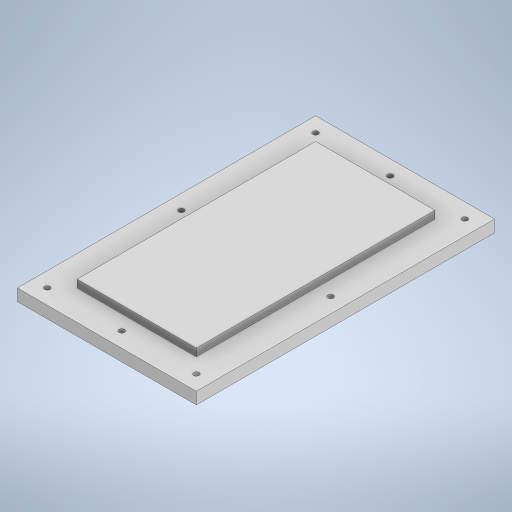
# Autodesk Inventor part: Faceplate
Saved by Autodesk Inventor 2024 (Build 280153020, 153B)
## iProperties
Created: 2023-07-16
Part Number: Faceplate
Material: Generic
Document SubType Name: Modeling
Designer: torban
Density: 1 g/cm^3
Appearance: Default
Author: torban
Autodesk Inventor part; units mm, degrees
ref_plane "YZ Plane" through (0, 0, 0) normal (1, 0, 0) x (0, 1, 0)
ref_plane "XZ Plane" through (0, 0, 0) normal (0, 1, 0) x (-1, 0, 0)
ref_plane "XY Plane" through (0, 0, 0) normal (0, 0, 1) x (1, 0, 0)
sketch "Sketch1" plane through (0, 0, 0) normal (0, 1, 0) x (-1, 0, 0)
  line L0 (0, 0) -> (100, 0)
  line L1 (100, 0) -> (100, -200)
  line L2 (100, -200) -> (0, -200)
  line L3 (0, -200) -> (0, 0)
  dimension "d0" = 200
  dimension "d1" = 100
  constraints: 8 end point, 2 parallel, 1 horizontal, 1 perpendicular
  measures "d0" distance of L0.end L1.end
  measures "d1" distance of L1.end L2.end
extrude "Extrusion1" add sketch "Sketch1" along normal blind 6.35
sketch "Sketch2" plane through (0, 0, 0) normal (0, -1, 0) x (1, 0, 0)
  line L0 (0, 0) -> (0, -200) projected
  line L1 (0, -200) -> (-100, -200) projected
  line L2 (-100, -200) -> (-100, 0) projected
  line L3 (-100, 0) -> (0, 0) projected
  line L4 (25, 25) -> (25, -225)
  line L5 (25, -225) -> (-125, -225)
  line L6 (-125, -225) -> (-125, 25)
  line L7 (-125, 25) -> (25, 25)
  dimension "d4" = 25
  constraints: 8 end point, 3 other
  measures "d4" distance between parallel lines of L3 L7
extrude "Extrusion2" add sketch "Sketch2" along normal blind 10 contours L0 L1 L2 L3 | L4 L5 L6 L7
sketch "Sketch3" plane through (0, 0, 0) normal (0, 1, 0) x (1, 0, 0)
  line L0 (-125, -25) -> (-125, 225) projected
  line L1 (-125, 225) -> (25, 225) projected
  line L2 (25, 225) -> (25, -25) projected
  line L3 (25, -25) -> (-125, -25) projected
  line L4 (0, 0) -> (0, 200) projected
  line L5 (0, 200) -> (-100, 200) projected
  line L6 (-100, 200) -> (-100, 0) projected
  line L7 (-100, 0) -> (0, 0) projected
  line L8 (12.5, -12.5) -> (12.5, 212.5)
  line L9 (12.5, 212.5) -> (-112.5, 212.5)
  line L10 (-112.5, 212.5) -> (-112.5, -12.5)
  line L11 (-112.5, -12.5) -> (12.5, -12.5)
  point P0 (12.5, 100)
  point P1 (-112.5, 100)
  point P2 (-50, 212.5)
  point P3 (-50, -12.5)
  dimension "d7" = 12.5
  constraints: 8 end point, 4 coincident, 4 midpoint, 3 other
  measures "d7" distance between parallel lines of L7 L11
hole "Hole1" at (-112.5, 0, 12.5) at (12.5, 0, 12.5) at (-112.5, 0, -212.5) at (12.5, 0, -212.5) at (12.5, 0, -100) at (-112.5, 0, -100) at (-50, 0, -212.5) at (-50, 0, 12.5) direction (0, -1, 0) diameter 4.69 end through all
body "Solid1"
